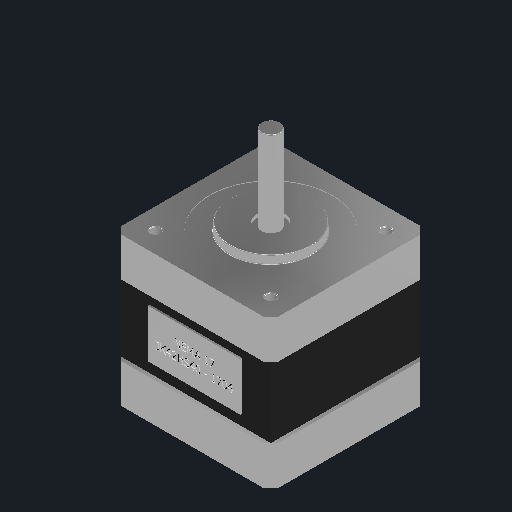
# Autodesk Inventor part: NEMA17
Saved by Autodesk Inventor 2024.2 (Build 282272000, 272)
## iProperties
Created: 2023-09-02
Part Number: NEMA17
Material: Genérico
Document SubType Name: Modeling
Designer: USUARIO
Density: 1 g/cm^3
Appearance: Valor por defecto
Author: USUARIO
Autodesk Inventor part; units mm, degrees
ref_plane "YZ Plane" through (0, 0, 0) normal (1, 0, 0) x (0, 1, 0)
sketch "Boceto1" plane through (0, 0, 0) normal (0, 1, 0) x (-1, 0, 0)
  line L0 (2, 0) -> (40.3, 0)
  line L1 (42.3, -2) -> (42.3, -40.3)
  line L2 (40.3, -42.3) -> (2, -42.3)
  line L3 (0, -40.3) -> (0, -2)
  line L4 (40.3, 0) -> (42.3, -2)
  line L5 (40.3, -42.3) -> (42.3, -40.3)
  line L6 (0, -40.3) -> (2, -42.3)
  line L7 (0, -2) -> (2, 0)
  point P0 (0, 0)
  point P1 (42.3, -42.3)
  point P2 (42.3, 0)
  point P3 (0, -42.3)
  dimension "d0" = 42.3
  dimension "d1" = 42.3
  dimension "d2" = 2
  dimension "d3" = 2
  dimension "d4" = 2
  dimension "d5" = 2
  dimension "d6" = 2
  dimension "d7" = 2
  dimension "d8" = 2
  dimension "d9" = 2
  constraints: 16 end point, 8 point on line, 2 parallel, 1 horizontal, 1 perpendicular
  measures "d0" distance of point (42.3, -42.3) point (0, -42.3)
  measures "d1" distance of point (42.3, 0) point (42.3, -42.3)
  measures "d2" distance of L0.end point (42.3, 0)
  measures "d3" distance of L1.start point (42.3, 0)
  measures "d4" distance of L2.start point (42.3, -42.3)
  measures "d5" distance of L1.end point (42.3, -42.3)
  measures "d6" distance of L3.start point (0, -42.3)
  measures "d7" distance of L2.end point (0, -42.3)
  measures "d8" distance of L3.end point (0, 0)
  measures "d9" distance of L0.start point (0, 0)
extrude "Extrusión1" add sketch "Boceto1" along normal blind 40
sketch "Boceto2" plane through (0, 40, 0) normal (0, 1, 0) x (1, 0, 0)
  line L0 (-2, 42.3) -> (-40.3, 42.3) projected
  line L1 (-40.3, 42.3) -> (-42.3, 40.3) projected
  line L2 (-42.3, 40.3) -> (-42.3, 2) projected
  line L3 (-42.3, 2) -> (-40.3, 0) projected
  line L4 (-40.3, 0) -> (-2, 0) projected
  line L5 (-2, 0) -> (0, 2) projected
  line L6 (0, 2) -> (0, 40.3) projected
  line L7 (0, 40.3) -> (-2, 42.3) projected
  line L8 (-42.3, 40.3) -> (-42.3, 2) projected
  line L9 (-42.3, 21.15) -> (0, 21.15)
  line L10 (-40.3, 0) -> (-2, 0) projected
  line L11 (-21.15, 0) -> (-21.15, 42.3)
  circle A0 centre (-21.15, 21.15) radius 11
  circle A1 centre (-36.65, 5.65) radius 1.25
  circle A2 centre (-36.65, 36.65) radius 1.25
  circle A3 centre (-5.65, 36.65) radius 1.25
  circle A4 centre (-5.65, 5.65) radius 1.25
  circle A5 centre (-21.15, 21.15) radius 2.5
  circle A6 centre (-21.15, 21.15) radius 16.5
  point P0 (0, 0)
  dimension "d12" = 22
  dimension "d13" = 2.5
  dimension "d14" = 2.5
  dimension "d15" = 2.5
  dimension "d16" = 2.5
  dimension "d17" = 31
  dimension "d18" = 31
  dimension "d19" = 5
  dimension "d63" = 33
  constraints: 7 centre point, 5 midpoint, 4 end point, 4 symmetric about line, 2 coincident
  measures "d12" diameter of A0
  measures "d13" diameter of A1
  measures "d14" diameter of A2
  measures "d15" diameter of A3
  measures "d16" diameter of A4
  measures "d17" distance of A2.centre A1.centre
  measures "d18" distance of A3.centre A2.centre
  measures "d19" diameter of A5
  measures "d63" diameter of A6
extrude "Extrusión2" add sketch "Boceto2" along normal blind 2 contours A0 L9 A5 L11 | L11 A5 L9 A0 | A0 L11 A5 L9 | L9 A5 L11 A0
extrude "Extrusión3" add sketch "Boceto2" along normal blind 24 contours A5 L9 L11 | L11 L9 A5 | L11 A5 L9 | L9 A5 L11
hole "Agujero1" at (-36.65, 40, -5.65) at (-36.65, 40, -36.65) at (-5.65, 40, -36.65) at (-5.65, 40, -5.65) direction (0, -1, 0) diameter 2.5 depth 4.5 tip angle 118 countersink diameter 3 countersink angle 90
sketch "Boceto5" plane through (0, 0, -2) normal (1, 0, 0) x (0, 0, -1)
  line L0 (0, 0) -> (38.3, 0) projected
  line L1 (38.3, 0) -> (38.3, 40) projected
  line L2 (0, 40) -> (38.3, 40) projected
  line L3 (0, 0) -> (0, 40) projected
  line L4 (0, 0) -> (0, 40) projected
  line L5 (0, 20) -> (38.3, 20)
  line L6 (38.3, 40) -> (0, 40) projected
  line L7 (19.15, 40) -> (19.15, 0)
  line L8 (38.3, 0) -> (0, 0) projected
  line L9 (40.3, 0) -> (40.3, 40) projected
  line L10 (-2, 10.5) -> (40.3, 10.5)
  line L11 (40.3, 10.5) -> (40.3, 29.5)
  line L12 (40.3, 29.5) -> (-2, 29.5)
  line L13 (-2, 29.5) -> (-2, 10.5)
  line L14 (-2, 10.5) -> (40.3, 29.5) construction
  line L15 (40.3, 10.5) -> (-2, 29.5) construction
  point P0 (-2, 0)
  point P1 (19.15, 20)
  dimension "d36" = 19
  constraints: 16 end point, 7 midpoint, 2 parallel, 1 horizontal, 1 perpendicular, 1 point on line
  measures "d36" distance of L11.end L10.end
extrude "Extrusión4" cut sketch "Boceto5" against normal blind 1 contours L10 L13 L12 L3 | L3 L5 L7 L10 | L7 L5 L1 L10 | L3 L12 L7 L5 | L1 L12 L9 L10 | L7 L12 L1 L5
ref_plane "Plano de trabajo2" through (-21.15, 0, -40.3) normal (-1, 0, 0) x (0, 0, 1)
mirror "Simetría1" about plane through (-21.15, 0, -40.3) normal (-1, 0, 0) of "Extrusión4"
sketch "Boceto6" plane through (-40.3, 0, 0) normal (0, 0, 1) x (1, 0, 0)
  line L0 (-1, 29.5) -> (-1, 10.5) projected
  line L1 (39.3, 10.5) -> (39.3, 29.5) projected
  line L2 (-1, 29.5) -> (-2, 29.5) projected
  line L3 (-1, 29.5) -> (39.3, 29.5)
  line L4 (39.3, 29.5) -> (39.3, 10.5)
  line L5 (39.3, 10.5) -> (-1, 10.5)
  line L6 (-1, 10.5) -> (-1, 29.5)
  point P0 (40.3, 0)
  constraints: 8 end point, 2 parallel, 1 horizontal, 1 perpendicular
extrude "Extrusión5" cut sketch "Boceto6" against normal blind 1
ref_plane "Plano de trabajo3" through (-2, 0, -21.15) normal (0, 0, -1) x (-1, 0, 0)
mirror "Simetría2" about plane through (-2, 0, -21.15) normal (0, 0, -1) of "Extrusión5"
sketch "Boceto7" plane through (-42.3, 0, -40.3) normal (-1, 0, 0) x (0, 0, 1)
  line L0 (0, 40) -> (38.3, 40) projected
  line L1 (0, 0) -> (38.3, 0) projected
  line L2 (19.15, 40) -> (19.15, 0)
  line L3 (38.3, 0) -> (0, 0) projected
  line L4 (15.15, 1) -> (23.15, 1)
  line L5 (23.15, 1) -> (23.15, 8)
  line L6 (23.15, 8) -> (15.15, 8)
  line L7 (15.15, 8) -> (15.15, 1)
  line L8 (15.15, 1) -> (23.15, 8) construction
  line L9 (23.15, 1) -> (15.15, 8) construction
  point P0 (40.3, 0)
  point P1 (19.15, 4.5)
  dimension "d41" = 8
  dimension "d42" = 7
  dimension "d43" = 1
  constraints: 14 end point, 4 midpoint, 2 parallel, 1 horizontal, 1 perpendicular, 1 point on line
  measures "d41" distance of L6.end L5.end
  measures "d42" distance of L5.end L4.end
  measures "d43" distance between parallel lines of L1 L4
extrude "Extrusión6" cut sketch "Boceto7" against normal blind 2
sketch "Boceto8" plane through (-40.3, 0, -40.3) normal (-1, 0, 0) x (0, 0, 1)
  line L0 (15.15, 1) -> (15.15, 8) projected
  line L1 (23.15, 8) -> (23.15, 1) projected
  line L2 (15.15, 8) -> (23.15, 8) projected
  line L3 (23.15, 1) -> (15.15, 1) projected
  line L4 (15.15, 1) -> (15.15, 8) projected
  line L5 (15.15, 4.5) -> (23.15, 4.5) construction
  line L6 (23.15, 8) -> (23.15, 1) projected
  circle A0 centre (16.15, 4.5) radius 0.5
  circle A1 centre (18.15, 4.5) radius 0.5
  circle A2 centre (20.15, 4.5) radius 0.5
  circle A3 centre (22.15, 4.5) radius 0.5
  point P0 (40.3, 0)
  dimension "d46" = 1
  dimension "d49" = 2
  dimension "d54" = 1
  constraints: 4 centre point, 2 end point, 2 midpoint, 1 horizontal, 1 point on line, 6 other
  measures "d46" diameter of A0
  measures "d49" distance of A0.centre A1.centre
  measures "d54" distance from line of L0 A0.centre
extrude "Extrusión7" add sketch "Boceto8" along normal blind 10 contours A0 | A1 | A2 | A3
sketch "Boceto9" plane through (-40.3, 0, -1) normal (0, 0, 1) x (1, 0, 0)
  line L0 (-1, 29.5) -> (-1, 10.5) projected
  line L1 (39.3, 10.5) -> (-1, 10.5) projected
  line L2 (39.3, 10.5) -> (39.3, 29.5) projected
  line L3 (-1, 29.5) -> (39.3, 29.5) projected
  line L4 (-1, 10.5) -> (-1, 29.5) projected
  line L5 (-1, 20) -> (39.3, 20) construction
  line L6 (39.3, 29.5) -> (39.3, 10.5) projected
  line L7 (6.65, 13.5) -> (31.65, 13.5)
  line L8 (31.65, 13.5) -> (31.65, 26.5)
  line L9 (31.65, 26.5) -> (6.65, 26.5)
  line L10 (6.65, 26.5) -> (6.65, 13.5)
  line L11 (6.65, 13.5) -> (31.65, 26.5) construction
  line L12 (31.65, 13.5) -> (6.65, 26.5) construction
  point P0 (40.3, 0)
  point P1 (19.15, 20)
  dimension "d57" = 25
  dimension "d58" = 13
  constraints: 14 end point, 5 midpoint, 2 parallel, 1 horizontal, 1 perpendicular
  measures "d57" distance of L9.end L8.end
  measures "d58" distance of L8.end L7.end
extrude "Extrusión8" add sketch "Boceto9" along normal blind 0.5 contours L10 L9 L8 L7
sketch "Boceto10" plane through (-40.3, 0, -0.5) normal (0, 0, 1) x (1, 0, 0)
  line L0 (31.65, 13.5) -> (31.65, 26.5) projected
  line L1 (31.65, 26.5) -> (6.65, 26.5) projected
  line L2 (6.65, 26.5) -> (6.65, 13.5) projected
  line L3 (6.65, 13.5) -> (31.65, 13.5) projected
  line L4 (6.65, 26.5) -> (6.65, 13.5) projected
  line L5 (6.65, 20) -> (31.65, 20) construction
  line L6 (31.65, 13.5) -> (31.65, 26.5) projected
  line L7 (8.2881, 22.6824) -> (30.0119, 22.6824) construction
  line L8 (30.0119, 22.6824) -> (30.0119, 17.3176) construction
  line L9 (30.0119, 17.3176) -> (8.2881, 17.3176) construction
  line L10 (8.2881, 17.3176) -> (8.2881, 22.6824) construction
  line L11 (31.65, 26.5) -> (6.65, 26.5) projected
  line L12 (19.15, 26.5) -> (19.15, 13.5) construction
  line L13 (6.65, 13.5) -> (31.65, 13.5) projected
  line L14 (15.2788, 20.6759) -> (14.9806, 20.6759)
  line L15 (14.9806, 20.6759) -> (14.0957, 22.4004)
  line L16 (14.0957, 22.4004) -> (14.0957, 20.6759)
  line L17 (14.0957, 20.6759) -> (13.8477, 20.6759)
  line L18 (13.8477, 20.6759) -> (13.8477, 22.6759)
  line L19 (13.8477, 22.6759) -> (14.2254, 22.6759)
  line L20 (14.2254, 22.6759) -> (15.0309, 21.0924)
  line L21 (15.0309, 21.0924) -> (15.0309, 22.6759)
  line L22 (15.0309, 22.6759) -> (15.2788, 22.6759)
  line L23 (15.2788, 22.6759) -> (15.2788, 20.6759)
  line L24 (15.684, 20.6759) -> (15.684, 22.6759)
  line L25 (15.684, 22.6759) -> (16.9353, 22.6759)
  line L26 (16.9353, 22.6759) -> (16.9353, 22.4393)
  line L27 (16.9353, 22.4393) -> (15.9498, 22.4393)
  line L28 (15.9498, 22.4393) -> (15.9498, 21.8914)
  line L29 (15.9498, 21.8914) -> (16.8688, 21.8914)
  line L30 (16.8688, 21.8914) -> (16.8688, 21.6548)
  line L31 (16.8688, 21.6548) -> (15.9498, 21.6548)
  line L32 (15.9498, 21.6548) -> (15.9498, 20.9125)
  line L33 (15.9498, 20.9125) -> (16.9353, 20.9125)
  line L34 (16.9353, 20.9125) -> (16.9353, 20.6759)
  line L35 (16.9353, 20.6759) -> (15.684, 20.6759)
  line L36 (18.9417, 20.6759) -> (18.6759, 20.6759)
  line L37 (18.6759, 20.6759) -> (18.6759, 22.3987)
  line L38 (18.6759, 22.3987) -> (18.1541, 21.2269)
  line L39 (18.1541, 21.2269) -> (17.992, 21.2269)
  line L40 (17.992, 21.2269) -> (17.475, 22.3987)
  line L41 (17.475, 22.3987) -> (17.475, 20.6759)
  line L42 (17.475, 20.6759) -> (17.227, 20.6759)
  line L43 (17.227, 20.6759) -> (17.227, 22.6759)
  line L44 (17.227, 22.6759) -> (17.59, 22.6759)
  line L45 (17.59, 22.6759) -> (18.0892, 21.5624)
  line L46 (18.0892, 21.5624) -> (18.5722, 22.6759)
  line L47 (18.5722, 22.6759) -> (18.9417, 22.6759)
  line L48 (18.9417, 22.6759) -> (18.9417, 20.6759)
  line L49 (19.1314, 20.6759) -> (19.8056, 22.6759)
  line L50 (19.8056, 22.6759) -> (20.133, 22.6759)
  line L51 (20.133, 22.6759) -> (20.8072, 20.6759)
  line L52 (20.8072, 20.6759) -> (20.5268, 20.6759)
  line L53 (20.5268, 20.6759) -> (20.3453, 21.235)
  line L54 (20.3453, 21.235) -> (19.5819, 21.235)
  line L55 (19.5819, 21.235) -> (19.4004, 20.6759)
  line L56 (19.4004, 20.6759) -> (19.1314, 20.6759)
  line L57 (20.2724, 21.4619) -> (19.9628, 22.4036)
  line L58 (19.9628, 22.4036) -> (19.6549, 21.4619)
  line L59 (19.6549, 21.4619) -> (20.2724, 21.4619)
  line L60 (22.932, 20.6759) -> (21.9563, 20.6759)
  line L61 (21.9563, 20.6759) -> (21.9563, 20.8801)
  line L62 (21.9563, 20.8801) -> (22.3194, 20.8801)
  line L63 (22.3194, 20.8801) -> (22.3194, 22.2205)
  line L64 (22.3194, 22.2205) -> (21.9563, 22.2205)
  line L65 (21.9563, 22.2205) -> (21.9563, 22.4036)
  spline S0 degree 2 poles (21.9563, 22.4036) (22.1622, 22.4036) (22.3566, 22.5203) (22.3696, 22.6824) knots 0 0 0 1 2 2 2
  line L66 (22.3696, 22.6824) -> (22.5771, 22.6824)
  line L67 (22.5771, 22.6824) -> (22.5771, 20.8801)
  line L68 (22.5771, 20.8801) -> (22.932, 20.8801)
  line L69 (22.932, 20.8801) -> (22.932, 20.6759)
  line L70 (24.556, 22.376) -> (23.6905, 20.6759)
  line L71 (23.6905, 20.6759) -> (23.4053, 20.6759)
  line L72 (23.4053, 20.6759) -> (24.3194, 22.4409)
  line L73 (24.3194, 22.4409) -> (23.287, 22.4409)
  line L74 (23.287, 22.4409) -> (23.287, 22.6759)
  line L75 (23.287, 22.6759) -> (24.556, 22.6759)
  line L76 (24.556, 22.6759) -> (24.556, 22.376)
  spline S1 degree 2 poles (9.6686, 17.9032) (9.6686, 17.6406) (9.3477, 17.3554) (9.0771, 17.3554) knots 0 0 0 1 2 2 2
  spline S2 degree 2 poles (9.0771, 17.3554) (9.0122, 17.3554) (8.7967, 17.3781) (8.7237, 17.3943) knots 0 0 0 1 2 2 2
  line L77 (8.7237, 17.3943) -> (8.7237, 17.6504)
  line L78 (8.7237, 17.6504) -> (8.7383, 17.6504)
  spline S3 degree 2 poles (8.7383, 17.6504) (8.7934, 17.6309) (8.9571, 17.5855) (9.0414, 17.5855) knots 0 0 0 1 2 2 2
  spline S4 degree 2 poles (9.0414, 17.5855) (9.1646, 17.5855) (9.3121, 17.6423) (9.3461, 17.6941) knots 0 0 0 1 2 2 2
  spline S5 degree 2 poles (9.3461, 17.6941) (9.3834, 17.7476) (9.4028, 17.9032) (9.4028, 18.0053) knots 0 0 0 1 2 2 2
  line L79 (9.4028, 18.0053) -> (9.4028, 19.1706)
  line L80 (9.4028, 19.1706) -> (8.9798, 19.1706)
  line L81 (8.9798, 19.1706) -> (8.9798, 19.3829)
  line L82 (8.9798, 19.3829) -> (9.6686, 19.3829)
  line L83 (9.6686, 19.3829) -> (9.6686, 17.9032)
  line L84 (11.5195, 17.3829) -> (11.1743, 17.3829)
  line L85 (11.1743, 17.3829) -> (10.4434, 18.3132)
  line L86 (10.4434, 18.3132) -> (10.3267, 18.182)
  line L87 (10.3267, 18.182) -> (10.3267, 17.3829)
  line L88 (10.3267, 17.3829) -> (10.0609, 17.3829)
  line L89 (10.0609, 17.3829) -> (10.0609, 19.3829)
  line L90 (10.0609, 19.3829) -> (10.3267, 19.3829)
  line L91 (10.3267, 19.3829) -> (10.3267, 18.464)
  line L92 (10.3267, 18.464) -> (11.1468, 19.3829)
  line L93 (11.1468, 19.3829) -> (11.4709, 19.3829)
  line L94 (11.4709, 19.3829) -> (10.6427, 18.4899)
  line L95 (10.6427, 18.4899) -> (11.5195, 17.3829)
  line L96 (12.9085, 18.0701) -> (12.6703, 18.0701)
  line L97 (12.6703, 18.0701) -> (12.6703, 17.3829)
  line L98 (12.6703, 17.3829) -> (12.4126, 17.3829)
  line L99 (12.4126, 17.3829) -> (12.4126, 18.0701)
  line L100 (12.4126, 18.0701) -> (11.5293, 18.0701)
  line L101 (11.5293, 18.0701) -> (11.5293, 18.3521)
  line L102 (11.5293, 18.3521) -> (12.4239, 19.3829)
  line L103 (12.4239, 19.3829) -> (12.6703, 19.3829)
  line L104 (12.6703, 19.3829) -> (12.6703, 18.2857)
  line L105 (12.6703, 18.2857) -> (12.9085, 18.2857)
  line L106 (12.9085, 18.2857) -> (12.9085, 18.0701)
  line L107 (12.4126, 18.2857) -> (12.4126, 19.0669)
  line L108 (12.4126, 19.0669) -> (11.74, 18.2857)
  line L109 (11.74, 18.2857) -> (12.4126, 18.2857)
  line L110 (14.3558, 17.3829) -> (13.1224, 17.3829)
  line L111 (13.1224, 17.3829) -> (13.1224, 17.6666)
  spline S6 degree 2 poles (13.1224, 17.6666) (13.2553, 17.7914) (13.492, 18.0231) (13.6054, 18.1479) knots 0 0 0 1 2 2 2
  spline S7 degree 2 poles (13.6054, 18.1479) (13.834, 18.3991) (14.0009, 18.7006) (14.0009, 18.8611) knots 0 0 0 1 2 2 2
  spline S8 degree 2 poles (14.0009, 18.8611) (14.0009, 18.9453) (13.949, 19.0717) (13.902, 19.1123) knots 0 0 0 1 2 2 2
  spline S9 degree 2 poles (13.902, 19.1123) (13.855, 19.1528) (13.7318, 19.1933) (13.6573, 19.1933) knots 0 0 0 1 2 2 2
  spline S10 degree 2 poles (13.6573, 19.1933) (13.586, 19.1933) (13.4401, 19.1576) (13.3737, 19.1301) knots 0 0 0 1 2 2 2
  spline S11 degree 2 poles (13.3737, 19.1301) (13.3169, 19.1074) (13.2116, 19.0426) (13.1792, 19.0199) knots 0 0 0 1 2 2 2
  line L112 (13.1792, 19.0199) -> (13.1646, 19.0199)
  line L113 (13.1646, 19.0199) -> (13.1646, 19.3051)
  spline S12 degree 2 poles (13.1646, 19.3051) (13.2472, 19.3457) (13.5438, 19.4251) (13.6767, 19.4251) knots 0 0 0 1 2 2 2
  spline S13 degree 2 poles (13.6767, 19.4251) (13.9571, 19.4251) (14.2732, 19.1285) (14.2732, 18.8756) knots 0 0 0 1 2 2 2
  spline S14 degree 2 poles (14.2732, 18.8756) (14.2732, 18.7573) (14.2181, 18.5596) (14.1694, 18.4753) knots 0 0 0 1 2 2 2
  spline S15 degree 2 poles (14.1694, 18.4753) (14.1208, 18.3878) (13.9798, 18.216) (13.902, 18.1333) knots 0 0 0 1 2 2 2
  spline S16 degree 2 poles (13.902, 18.1333) (13.7756, 17.9956) (13.466, 17.7006) (13.3737, 17.6147) knots 0 0 0 1 2 2 2
  line L114 (13.3737, 17.6147) -> (14.3558, 17.6147)
  line L115 (14.3558, 17.6147) -> (14.3558, 17.3829)
  line L116 (16.1322, 17.3829) -> (15.8664, 17.3829)
  line L117 (15.8664, 17.3829) -> (15.8664, 18.3619)
  line L118 (15.8664, 18.3619) -> (14.9458, 18.3619)
  line L119 (14.9458, 18.3619) -> (14.9458, 17.3829)
  line L120 (14.9458, 17.3829) -> (14.68, 17.3829)
  line L121 (14.68, 17.3829) -> (14.68, 19.3829)
  line L122 (14.68, 19.3829) -> (14.9458, 19.3829)
  line L123 (14.9458, 19.3829) -> (14.9458, 18.5985)
  line L124 (14.9458, 18.5985) -> (15.8664, 18.5985)
  line L125 (15.8664, 18.5985) -> (15.8664, 19.3829)
  line L126 (15.8664, 19.3829) -> (16.1322, 19.3829)
  line L127 (16.1322, 19.3829) -> (16.1322, 17.3829)
  spline S17 degree 2 poles (17.0949, 17.3473) (16.8777, 17.3473) (16.573, 17.438) (16.4385, 17.5029) knots 0 0 0 1 2 2 2
  line L128 (16.4385, 17.5029) -> (16.4385, 17.8367)
  line L129 (16.4385, 17.8367) -> (16.4579, 17.8367)
  spline S18 degree 2 poles (16.4579, 17.8367) (16.5892, 17.7136) (16.9215, 17.5774) (17.0754, 17.5774) knots 0 0 0 1 2 2 2
  spline S19 degree 2 poles (17.0754, 17.5774) (17.2959, 17.5774) (17.5212, 17.7606) (17.5212, 17.9113) knots 0 0 0 1 2 2 2
  spline S20 degree 2 poles (17.5212, 17.9113) (17.5212, 18.0312) (17.4028, 18.1803) (17.2748, 18.2176) knots 0 0 0 1 2 2 2
  spline S21 degree 2 poles (17.2748, 18.2176) (17.1824, 18.2435) (17.0284, 18.2792) (16.9134, 18.3084) knots 0 0 0 1 2 2 2
  spline S22 degree 2 poles (16.9134, 18.3084) (16.8096, 18.3359) (16.6459, 18.4186) (16.5827, 18.485) knots 0 0 0 1 2 2 2
  spline S23 degree 2 poles (16.5827, 18.485) (16.5212, 18.5515) (16.4531, 18.7298) (16.4531, 18.8465) knots 0 0 0 1 2 2 2
  spline S24 degree 2 poles (16.4531, 18.8465) (16.4531, 19.0896) (16.8323, 19.4186) (17.1257, 19.4186) knots 0 0 0 1 2 2 2
  spline S25 degree 2 poles (17.1257, 19.4186) (17.2942, 19.4186) (17.5925, 19.3521) (17.7205, 19.2889) knots 0 0 0 1 2 2 2
  line L130 (17.7205, 19.2889) -> (17.7205, 18.9713)
  line L131 (17.7205, 18.9713) -> (17.7011, 18.9713)
  spline S26 degree 2 poles (17.7011, 18.9713) (17.6054, 19.0588) (17.3072, 19.1884) (17.1435, 19.1884) knots 0 0 0 1 2 2 2
  spline S27 degree 2 poles (17.1435, 19.1884) (16.9588, 19.1884) (16.7302, 19.015) (16.7302, 18.874) knots 0 0 0 1 2 2 2
  spline S28 degree 2 poles (16.7302, 18.874) (16.7302, 18.7476) (16.8647, 18.5969) (16.9912, 18.5628) knots 0 0 0 1 2 2 2
  spline S29 degree 2 poles (16.9912, 18.5628) (17.0754, 18.5401) (17.3202, 18.4818) (17.4012, 18.4575) knots 0 0 0 1 2 2 2
  spline S30 degree 2 poles (17.4012, 18.4575) (17.607, 18.3943) (17.7983, 18.1398) (17.7983, 17.9534) knots 0 0 0 1 2 2 2
  spline S31 degree 2 poles (17.7983, 17.9534) (17.7983, 17.8351) (17.7027, 17.6082) (17.6168, 17.5288) knots 0 0 0 1 2 2 2
  spline S32 degree 2 poles (17.6168, 17.5288) (17.5212, 17.4413) (17.278, 17.3473) (17.0949, 17.3473) knots 0 0 0 1 2 2 2
  line L132 (19.2991, 18.0701) -> (19.0609, 18.0701)
  line L133 (19.0609, 18.0701) -> (19.0609, 17.3829)
  line L134 (19.0609, 17.3829) -> (18.8032, 17.3829)
  line L135 (18.8032, 17.3829) -> (18.8032, 18.0701)
  line L136 (18.8032, 18.0701) -> (17.9199, 18.0701)
  line L137 (17.9199, 18.0701) -> (17.9199, 18.3521)
  line L138 (17.9199, 18.3521) -> (18.8145, 19.3829)
  line L139 (18.8145, 19.3829) -> (19.0609, 19.3829)
  line L140 (19.0609, 19.3829) -> (19.0609, 18.2857)
  line L141 (19.0609, 18.2857) -> (19.2991, 18.2857)
  line L142 (19.2991, 18.2857) -> (19.2991, 18.0701)
  line L143 (18.8032, 18.2857) -> (18.8032, 19.0669)
  line L144 (18.8032, 19.0669) -> (18.1306, 18.2857)
  line L145 (18.1306, 18.2857) -> (18.8032, 18.2857)
  spline S33 degree 2 poles (20.7578, 18.3829) (20.7578, 17.8448) (20.445, 17.3408) (20.1192, 17.3408) knots 0 0 0 1 2 2 2
  spline S34 degree 2 poles (20.1192, 17.3408) (19.7886, 17.3408) (19.479, 17.8546) (19.479, 18.3813) knots 0 0 0 1 2 2 2
  spline S35 degree 2 poles (19.479, 18.3813) (19.479, 18.9226) (19.7918, 19.4235) (20.1192, 19.4235) knots 0 0 0 1 2 2 2
  spline S36 degree 2 poles (20.1192, 19.4235) (20.4482, 19.4235) (20.7578, 18.9048) (20.7578, 18.3829) knots 0 0 0 1 2 2 2
  spline S37 degree 2 poles (20.4142, 17.7735) (20.4531, 17.8724) (20.4855, 18.1771) (20.4855, 18.3829) knots 0 0 0 1 2 2 2
  spline S38 degree 2 poles (20.4855, 18.3829) (20.4855, 18.5888) (20.4531, 18.8918) (20.4126, 18.994) knots 0 0 0 1 2 2 2
  spline S39 degree 2 poles (20.4126, 18.994) (20.372, 19.0961) (20.231, 19.2014) (20.1192, 19.2014) knots 0 0 0 1 2 2 2
  spline S40 degree 2 poles (20.1192, 19.2014) (20.0074, 19.2014) (19.8631, 19.0961) (19.821, 18.9907) knots 0 0 0 1 2 2 2
  spline S41 degree 2 poles (19.821, 18.9907) (19.7805, 18.8886) (19.7513, 18.5774) (19.7513, 18.3813) knots 0 0 0 1 2 2 2
  spline S42 degree 2 poles (19.7513, 18.3813) (19.7513, 18.1706) (19.7772, 17.8886) (19.8194, 17.7784) knots 0 0 0 1 2 2 2
  spline S43 degree 2 poles (19.8194, 17.7784) (19.8583, 17.6747) (20.0025, 17.5628) (20.1192, 17.5628) knots 0 0 0 1 2 2 2
  spline S44 degree 2 poles (20.1192, 17.5628) (20.2294, 17.5628) (20.3737, 17.6682) (20.4142, 17.7735) knots 0 0 0 1 2 2 2
  line L146 (22.6054, 18.1366) -> (21.8485, 18.1366)
  line L147 (21.8485, 18.1366) -> (21.8485, 18.3797)
  line L148 (21.8485, 18.3797) -> (22.6054, 18.3797)
  line L149 (22.6054, 18.3797) -> (22.6054, 18.1366)
  line L150 (24.8631, 17.3829) -> (23.8874, 17.3829)
  line L151 (23.8874, 17.3829) -> (23.8874, 17.5871)
  line L152 (23.8874, 17.5871) -> (24.2505, 17.5871)
  line L153 (24.2505, 17.5871) -> (24.2505, 18.9275)
  line L154 (24.2505, 18.9275) -> (23.8874, 18.9275)
  line L155 (23.8874, 18.9275) -> (23.8874, 19.1106)
  spline S45 degree 2 poles (23.8874, 19.1106) (24.0933, 19.1106) (24.2878, 19.2273) (24.3007, 19.3894) knots 0 0 0 1 2 2 2
  line L156 (24.3007, 19.3894) -> (24.5082, 19.3894)
  line L157 (24.5082, 19.3894) -> (24.5082, 17.5871)
  line L158 (24.5082, 17.5871) -> (24.8631, 17.5871)
  line L159 (24.8631, 17.5871) -> (24.8631, 17.3829)
  line L160 (26.4871, 19.0831) -> (25.6216, 17.3829)
  line L161 (25.6216, 17.3829) -> (25.3364, 17.3829)
  line L162 (25.3364, 17.3829) -> (26.2505, 19.1479)
  line L163 (26.2505, 19.1479) -> (25.2181, 19.1479)
  line L164 (25.2181, 19.1479) -> (25.2181, 19.3829)
  line L165 (25.2181, 19.3829) -> (26.4871, 19.3829)
  line L166 (26.4871, 19.3829) -> (26.4871, 19.0831)
  spline S46 degree 2 poles (27.9766, 18.3829) (27.9766, 17.8448) (27.6638, 17.3408) (27.338, 17.3408) knots 0 0 0 1 2 2 2
  spline S47 degree 2 poles (27.338, 17.3408) (27.0074, 17.3408) (26.6978, 17.8546) (26.6978, 18.3813) knots 0 0 0 1 2 2 2
  spline S48 degree 2 poles (26.6978, 18.3813) (26.6978, 18.9226) (27.0106, 19.4235) (27.338, 19.4235) knots 0 0 0 1 2 2 2
  spline S49 degree 2 poles (27.338, 19.4235) (27.667, 19.4235) (27.9766, 18.9048) (27.9766, 18.3829) knots 0 0 0 1 2 2 2
  spline S50 degree 2 poles (27.633, 17.7735) (27.6719, 17.8724) (27.7043, 18.1771) (27.7043, 18.3829) knots 0 0 0 1 2 2 2
  spline S51 degree 2 poles (27.7043, 18.3829) (27.7043, 18.5888) (27.6719, 18.8918) (27.6314, 18.994) knots 0 0 0 1 2 2 2
  spline S52 degree 2 poles (27.6314, 18.994) (27.5908, 19.0961) (27.4498, 19.2014) (27.338, 19.2014) knots 0 0 0 1 2 2 2
  spline S53 degree 2 poles (27.338, 19.2014) (27.2262, 19.2014) (27.0819, 19.0961) (27.0398, 18.9907) knots 0 0 0 1 2 2 2
  spline S54 degree 2 poles (27.0398, 18.9907) (26.9993, 18.8886) (26.9701, 18.5774) (26.9701, 18.3813) knots 0 0 0 1 2 2 2
  spline S55 degree 2 poles (26.9701, 18.3813) (26.9701, 18.1706) (26.996, 17.8886) (27.0382, 17.7784) knots 0 0 0 1 2 2 2
  spline S56 degree 2 poles (27.0382, 17.7784) (27.0771, 17.6747) (27.2213, 17.5628) (27.338, 17.5628) knots 0 0 0 1 2 2 2
  spline S57 degree 2 poles (27.338, 17.5628) (27.4482, 17.5628) (27.5925, 17.6682) (27.633, 17.7735) knots 0 0 0 1 2 2 2
  line L167 (29.5195, 18.0701) -> (29.2813, 18.0701)
  line L168 (29.2813, 18.0701) -> (29.2813, 17.3829)
  line L169 (29.2813, 17.3829) -> (29.0236, 17.3829)
  line L170 (29.0236, 17.3829) -> (29.0236, 18.0701)
  line L171 (29.0236, 18.0701) -> (28.1403, 18.0701)
  line L172 (28.1403, 18.0701) -> (28.1403, 18.3521)
  line L173 (28.1403, 18.3521) -> (29.0349, 19.3829)
  line L174 (29.0349, 19.3829) -> (29.2813, 19.3829)
  line L175 (29.2813, 19.3829) -> (29.2813, 18.2857)
  line L176 (29.2813, 18.2857) -> (29.5195, 18.2857)
  line L177 (29.5195, 18.2857) -> (29.5195, 18.0701)
  line L178 (29.0236, 18.2857) -> (29.0236, 19.0669)
  line L179 (29.0236, 19.0669) -> (28.351, 18.2857)
  line L180 (28.351, 18.2857) -> (29.0236, 18.2857)
  point P0 (40.3, 0)
  constraints: 4 end point, 4 midpoint, 4 other
extrude "Extrusión9" cut sketch "Boceto10" against normal blind 0.2 contours L14 L15 L16 L17 L18 L19 L20 L21 L22 L23 | L24 L25 L26 L27 L28 L29 L30 L31 L32 L33 L34 L35 | L36 L37 L38 L39 L40 L41 L42 L43 L44 L45 L46 L47 L48 | L49 L50 L51 L52 L53 L54 L55 L56 | L60 L61 L62 L63 L64 L65 S0 L66 L67 L68 L69 | L70 L71 L72 L73 L74 L75 L76 | S1 S2 L77 L78 S3 S4 S5 L79 L80 L81 L82 L83 | L84 L85 L86 L87 L88 L89 L90 L91 L92 L93 L94 L95 | L96 L97 L98 L99 L100 L101 L102 L103 L104 L105 L106 | L110 L111 S6 S7 S8 S9 S10 S11 L112 L113 S12 S13 S14 S15 S16 L114 L115 | L116 L117 L118 L119 L120 L121 L122 L123 L124 L125 L126 L127 | S17 L128 L129 S18 S19 S20 S21 S22 S23 S24 S25 L130 L131 S26 S27 S28 S29 S30 S31 S32 | L132 L133 L134 L135 L136 L137 L138 L139 L140 L141 L142 | S33 S34 S35 S36 | L146 L147 L148 L149 | L150 L151 L152 L153 L154 L155 S45 L156 L157 L158 L159 | L160 L161 L162 L163 L164 L165 L166 | S46 S47 S48 S49 | L167 L168 L169 L170 L171 L172 L173 L174 L175 L176 L177
extrude "Extrusión10" cut sketch "Boceto2" against normal blind 0.2 contours A6 L9 A0 L11 | L11 A0 L9 A6 | A6 L11 A0 L9 | L9 A0 L11 A6
fillet "Empalme1" radius 0.2 1 edges at (-32.15, 39.8, -21.15)
sketch "Boceto11" plane through (-21.15, 42, -21.15) normal (0, 1, 0) x (1, 0, 0)
  circle A0 centre (0, 0) radius 2.5 projected
  circle A1 centre (0, 0) radius 3.75
  point P0 (21.15, -21.15)
  dimension "d67" = 7.5
  constraints: 1 centre point, 1 coincident
  measures "d67" diameter of A1
extrude "Extrusión11" cut sketch "Boceto11" against normal blind 1
fillet "Empalme2" radius 0.2 1 edges at (-23.65, 64, -21.15)
fillet "Empalme3" radius 0.2 1 edges at (-32.15, 42, -21.15)
sketch "Boceto12" plane through (0, 0, 0) normal (0, -1, 0) x (1, 0, 0)
  circle A0 centre (-21.15, -21.15) radius 3.75 projected
  line L0 (-2, -42.3) -> (-40.3, -42.3) projected
  line L1 (0, -40.3) -> (-2, -42.3) projected
  line L2 (0, -2) -> (0, -40.3) projected
  line L3 (-2, 0) -> (0, -2) projected
  line L4 (-40.3, 0) -> (-2, 0) projected
  line L5 (-42.3, -2) -> (-40.3, 0) projected
  line L6 (-42.3, -40.3) -> (-42.3, -2) projected
  line L7 (-40.3, -42.3) -> (-42.3, -40.3) projected
  circle A1 centre (-36.65, -5.65) radius 1.25 projected
  circle A2 centre (-36.65, -5.65) radius 1.25
  circle A3 centre (-5.65, -5.65) radius 1.25
  circle A4 centre (-36.65, -36.65) radius 1.25
  circle A5 centre (-5.65, -36.65) radius 1.25
  point P0 (0, 0)
  dimension "d74" = 31
  dimension "d77" = 31
  constraints: 4 centre point, 1 coincident, 1 horizontal, 1 vertical, 6 other
  measures "d74" distance of A2.centre A3.centre
  measures "d77" distance of A2.centre A4.centre
extrude "Extrusión12" cut sketch "Boceto12" against normal blind 1.5 contours A0
hole "Agujero2" at (-36.65, 0, -5.65) at (-5.65, 0, -5.65) at (-36.65, 0, -36.65) at (-5.65, 0, -36.65) direction (0, 1, 0) diameter 2.5 depth 4.5 tip angle 118 countersink diameter 3 countersink angle 90
thread "Rosca1" size "M2.5x0.45" class "6H" standard "ANSI Metric M Profile" full length
thread "Rosca2" size "M2.5x0.45" class "6H" standard "ANSI Metric M Profile" full length
thread "Rosca3" size "M2.5x0.45" class "6H" standard "ANSI Metric M Profile" full length
thread "Rosca4" size "M2.5x0.45" class "6H" standard "ANSI Metric M Profile" full length
thread "Rosca5" size "M2.5x0.45" class "6H" standard "ANSI Metric M Profile" full length
thread "Rosca6" size "M2.5x0.45" class "6H" standard "ANSI Metric M Profile" full length
thread "Rosca7" size "M2.5x0.45" class "6H" standard "ANSI Metric M Profile" full length
thread "Rosca8" size "M2.5x0.45" class "6H" standard "ANSI Metric M Profile" full length
equation "\"d3\" = d2"
equation "\"d4\" = d2"
equation "\"d5\" = d4"
equation "\"d6\" = d2"
equation "\"d7\" = d6"
equation "\"d8\" = d2"
equation "\"d9\" = d8"
